Autodesk Inventor part; units mm, degrees
(part 2 of 2)
sketch "Sketch9" plane through (-10, 21.48, -77.0624) normal (0, 0, -1) x (-1, 0, 0)
  line L0 (0.1006, 0.0497) -> (90.0454, 0.0497) construction
  line L1 (90.0454, 0.0497) -> (90.0454, -43.0368) construction
  line L2 (90.0454, -43.0368) -> (0.1006, -43.0368) construction
  line L3 (0.1006, -43.0368) -> (0.1006, 0.0497) construction
  line L4 (5.8424, -17.3579) -> (5.8424, -12.0619)
  line L5 (5.8424, -12.0619) -> (5.6332, -12.0619)
  spline S0 degree 2 poles (5.6332, -12.0619) (5.1253, -12.0619) (4.707, -11.6884) (4.707, -11.3821) knots 0 0 0 1 2 2 2
  spline S1 degree 2 poles (4.707, -11.3821) (4.707, -11.0833) (5.1253, -10.7099) (5.6332, -10.7099) knots 0 0 0 1 2 2 2
  line L6 (5.6332, -10.7099) -> (9.0245, -10.7099)
  spline S2 degree 2 poles (9.0245, -10.7099) (10.2345, -10.7099) (11.7135, -12.0619) (11.7135, -12.9956) knots 0 0 0 1 2 2 2
  spline S3 degree 2 poles (11.7135, -12.9956) (11.7135, -13.4363) (11.3699, -14.2206) (11.0263, -14.5493) knots 0 0 0 1 2 2 2
  spline S4 degree 2 poles (11.0263, -14.5493) (11.6687, -14.9302) (12.3036, -15.9536) (12.3036, -16.596) knots 0 0 0 1 2 2 2
  spline S5 degree 2 poles (12.3036, -16.596) (12.3036, -17.1114) (12.0721, -17.5521) knots 0 0 0 1 1 1
  spline S6 degree 2 poles (12.0721, -17.5521) (11.9003, -17.8882) (11.6538, -18.0824) knots 0 0 0 1 1 1
  spline S7 degree 2 poles (11.6538, -18.0824) (11.3176, -18.3588) (10.3391, -18.7099) (9.6071, -18.7099) knots 0 0 0 1 2 2 2
  line L7 (9.6071, -18.7099) -> (5.6332, -18.7099)
  spline S8 degree 2 poles (5.6332, -18.7099) (5.1253, -18.7099) (4.707, -18.3364) (4.707, -18.0301) knots 0 0 0 1 2 2 2
  spline S9 degree 2 poles (4.707, -18.0301) (4.707, -17.7239) (5.1253, -17.3579) (5.6332, -17.3579) knots 0 0 0 1 2 2 2
  line L8 (5.6332, -17.3579) -> (5.8424, -17.3579)
  line L9 (7.1944, -17.3579) -> (9.5324, -17.3579)
  spline S10 degree 2 poles (9.5324, -17.3579) (10.3541, -17.3579) (10.6977, -17.1114) knots 0 0 0 1 1 1
  spline S11 degree 2 poles (10.6977, -17.1114) (10.9516, -16.9321) (10.9516, -16.5885) knots 0 0 0 1 1 1
  spline S12 degree 2 poles (10.9516, -16.5885) (10.9516, -16.1851) (9.9358, -15.3933) (8.9871, -15.3933) knots 0 0 0 1 2 2 2
  line L10 (8.9871, -15.3933) -> (7.1944, -15.3933)
  line L11 (7.1944, -15.3933) -> (7.1944, -17.3579)
  line L12 (7.1944, -14.0413) -> (8.6809, -14.0413)
  spline S13 degree 2 poles (8.6809, -14.0413) (9.4801, -14.0413) (10.003, -13.638) knots 0 0 0 1 1 1
  spline S14 degree 2 poles (10.003, -13.638) (10.3615, -13.3616) (10.3615, -12.9582) knots 0 0 0 1 1 1
  spline S15 degree 2 poles (10.3615, -12.9582) (10.3615, -12.5997) (9.6893, -12.0619) (8.9572, -12.0619) knots 0 0 0 1 2 2 2
  line L13 (8.9572, -12.0619) -> (7.1944, -12.0619)
  line L14 (7.1944, -12.0619) -> (7.1944, -14.0413)
  line L15 (19.5791, -12.7192) -> (19.5791, -17.3579)
  spline S16 degree 2 poles (19.5791, -17.3579) (20.087, -17.3579) (20.5053, -17.7313) (20.5053, -18.0376) knots 0 0 0 1 2 2 2
  spline S17 degree 2 poles (20.5053, -18.0376) (20.5053, -18.3439) (20.087, -18.7099) (19.5791, -18.7099) knots 0 0 0 1 2 2 2
  line L16 (19.5791, -18.7099) -> (18.2271, -18.7099)
  line L17 (18.2271, -18.7099) -> (18.2271, -18.3961)
  spline S18 degree 2 poles (18.2271, -18.3961) (17.6444, -18.6576) (16.5912, -18.9265) (16.1132, -18.9265) knots 0 0 0 1 2 2 2
  spline S19 degree 2 poles (16.1132, -18.9265) (15.4484, -18.9265) (14.4698, -18.3663) (14.186, -17.8733) knots 0 0 0 1 2 2 2
  spline S20 degree 2 poles (14.186, -17.8733) (13.9843, -17.5147) (13.9843, -16.9769) knots 0 0 0 1 1 1
  line L18 (13.9843, -16.9769) -> (13.9843, -14.0712)
  line L19 (13.9843, -14.0712) -> (13.7528, -14.0712)
  spline S21 degree 2 poles (13.7528, -14.0712) (13.2448, -14.0712) (12.8265, -13.6977) (12.8265, -13.3915) knots 0 0 0 1 2 2 2
  spline S22 degree 2 poles (12.8265, -13.3915) (12.8265, -13.0852) (13.2448, -12.7192) (13.7528, -12.7192) knots 0 0 0 1 2 2 2
  line L20 (13.7528, -12.7192) -> (15.3363, -12.7192)
  line L21 (15.3363, -12.7192) -> (15.3363, -16.7453)
  spline S23 degree 2 poles (15.3363, -16.7453) (15.3363, -17.1711) (15.7546, -17.5745) (16.1804, -17.5745) knots 0 0 0 1 2 2 2
  spline S24 degree 2 poles (16.1804, -17.5745) (16.5912, -17.5745) (17.5324, -17.2533) (18.2271, -16.8275) knots 0 0 0 1 2 2 2
  line L22 (18.2271, -16.8275) -> (18.2271, -14.0712)
  line L23 (18.2271, -14.0712) -> (17.7416, -14.0712)
  spline S25 degree 2 poles (17.7416, -14.0712) (17.2336, -14.0712) (16.8153, -13.6977) (16.8153, -13.3915) knots 0 0 0 1 2 2 2
  spline S26 degree 2 poles (16.8153, -13.3915) (16.8153, -13.0852) (17.2336, -12.7192) (17.7416, -12.7192) knots 0 0 0 1 2 2 2
  line L24 (17.7416, -12.7192) -> (19.5791, -12.7192)
  line L25 (25.4801, -12.7192) -> (25.4801, -17.3579)
  line L26 (25.4801, -17.3579) -> (27.101, -17.3579)
  spline S27 degree 2 poles (27.101, -17.3579) (27.609, -17.3579) (28.0273, -17.7313) (28.0273, -18.0376) knots 0 0 0 1 2 2 2
  spline S28 degree 2 poles (28.0273, -18.0376) (28.0273, -18.3439) (27.609, -18.7099) (27.101, -18.7099) knots 0 0 0 1 2 2 2
  line L27 (27.101, -18.7099) -> (22.5072, -18.7099)
  spline S29 degree 2 poles (22.5072, -18.7099) (21.9993, -18.7099) (21.581, -18.3364) (21.581, -18.0301) knots 0 0 0 1 2 2 2
  spline S30 degree 2 poles (21.581, -18.0301) (21.581, -17.7239) (21.9993, -17.3579) (22.5072, -17.3579) knots 0 0 0 1 2 2 2
  line L28 (22.5072, -17.3579) -> (24.1281, -17.3579)
  line L29 (24.1281, -17.3579) -> (24.1281, -14.0712)
  line L30 (24.1281, -14.0712) -> (23.0375, -14.0712)
  spline S31 degree 2 poles (23.0375, -14.0712) (22.5296, -14.0712) (22.1113, -13.6977) (22.1113, -13.3915) knots 0 0 0 1 2 2 2
  spline S32 degree 2 poles (22.1113, -13.3915) (22.1113, -13.0852) (22.5296, -12.7192) (23.0375, -12.7192) knots 0 0 0 1 2 2 2
  line L31 (23.0375, -12.7192) -> (25.4801, -12.7192)
  line L32 (25.2934, -10.1571) -> (25.2934, -11.5913)
  line L33 (25.2934, -11.5913) -> (23.6874, -11.5913)
  line L34 (23.6874, -11.5913) -> (23.6874, -10.1571)
  line L35 (23.6874, -10.1571) -> (25.2934, -10.1571)
  line L36 (33.5847, -10.1571) -> (33.5847, -17.3579)
  line L37 (33.5847, -17.3579) -> (35.2056, -17.3579)
  spline S33 degree 2 poles (35.2056, -17.3579) (35.7135, -17.3579) (36.1318, -17.7313) (36.1318, -18.0376) knots 0 0 0 1 2 2 2
  spline S34 degree 2 poles (36.1318, -18.0376) (36.1318, -18.3439) (35.7135, -18.7099) (35.2056, -18.7099) knots 0 0 0 1 2 2 2
  line L38 (35.2056, -18.7099) -> (30.6118, -18.7099)
  spline S35 degree 2 poles (30.6118, -18.7099) (30.1038, -18.7099) (29.6855, -18.3364) (29.6855, -18.0301) knots 0 0 0 1 2 2 2
  spline S36 degree 2 poles (29.6855, -18.0301) (29.6855, -17.7239) (30.1038, -17.3579) (30.6118, -17.3579) knots 0 0 0 1 2 2 2
  line L39 (30.6118, -17.3579) -> (32.2327, -17.3579)
  line L40 (32.2327, -17.3579) -> (32.2327, -11.5091)
  line L41 (32.2327, -11.5091) -> (31.1421, -11.5091)
  spline S37 degree 2 poles (31.1421, -11.5091) (30.6342, -11.5091) (30.2159, -11.1356) (30.2159, -10.8294) knots 0 0 0 1 2 2 2
  spline S38 degree 2 poles (30.2159, -10.8294) (30.2159, -10.5231) (30.6342, -10.1571) (31.1421, -10.1571) knots 0 0 0 1 2 2 2
  line L42 (31.1421, -10.1571) -> (33.5847, -10.1571)
  line L43 (44.1169, -10.1571) -> (44.1169, -17.3579)
  line L44 (44.1169, -17.3579) -> (44.3485, -17.3579)
  spline S39 degree 2 poles (44.3485, -17.3579) (44.8564, -17.3579) (45.2747, -17.7313) (45.2747, -18.0376) knots 0 0 0 1 2 2 2
  spline S40 degree 2 poles (45.2747, -18.0376) (45.2747, -18.3439) (44.8564, -18.7099) (44.3485, -18.7099) knots 0 0 0 1 2 2 2
  line L45 (44.3485, -18.7099) -> (42.7649, -18.7099)
  line L46 (42.7649, -18.7099) -> (42.7649, -18.3812)
  spline S41 degree 2 poles (42.7649, -18.3812) (42.3018, -18.6501) (41.2934, -18.9265) (40.7556, -18.9265) knots 0 0 0 1 2 2 2
  spline S42 degree 2 poles (40.7556, -18.9265) (39.2392, -18.9265) (37.3793, -17.1636) (37.3793, -15.8565) knots 0 0 0 1 2 2 2
  spline S43 degree 2 poles (37.3793, -15.8565) (37.3793, -14.482) (39.3289, -12.5474) (40.7331, -12.5474) knots 0 0 0 1 2 2 2
  spline S44 degree 2 poles (40.7331, -12.5474) (41.256, -12.5474) (42.2719, -12.8686) (42.7649, -13.1973) knots 0 0 0 1 2 2 2
  line L47 (42.7649, -13.1973) -> (42.7649, -11.5091)
  line L48 (42.7649, -11.5091) -> (42.5333, -11.5091)
  spline S45 degree 2 poles (42.5333, -11.5091) (42.0254, -11.5091) (41.6071, -11.1431) (41.6071, -10.8368) knots 0 0 0 1 2 2 2
  spline S46 degree 2 poles (41.6071, -10.8368) (41.6071, -10.5306) (42.0254, -10.1571) (42.5333, -10.1571) knots 0 0 0 1 2 2 2
  line L49 (42.5333, -10.1571) -> (44.1169, -10.1571)
  spline S47 degree 2 poles (42.7649, -15.8938) (42.7649, -15.0572) (41.5922, -13.8994) (40.7481, -13.8994) knots 0 0 0 1 2 2 2
  spline S48 degree 2 poles (40.7481, -13.8994) (39.904, -13.8994) (38.7313, -15.0572) (38.7313, -15.8789) knots 0 0 0 1 2 2 2
  spline S49 degree 2 poles (38.7313, -15.8789) (38.7313, -16.6184) (39.7845, -17.5745) (40.7481, -17.5745) knots 0 0 0 1 2 2 2
  spline S50 degree 2 poles (40.7481, -17.5745) (41.6967, -17.5745) (42.7649, -16.6184) (42.7649, -15.8938) knots 0 0 0 1 2 2 2
  line L50 (50.3391, -18.7099) -> (50.3391, -18.3961)
  spline S51 degree 2 poles (50.3391, -18.3961) (49.8312, -18.6576) (48.6062, -18.9265) (48.1057, -18.9265) knots 0 0 0 1 2 2 2
  spline S52 degree 2 poles (48.1057, -18.9265) (47.0226, -18.9265) (45.6631, -17.7762) (45.6631, -17.0815) knots 0 0 0 1 2 2 2
  spline S53 degree 2 poles (45.6631, -17.0815) (45.6631, -16.2299) (47.3961, -14.7808) (48.9199, -14.7808) knots 0 0 0 1 2 2 2
  spline S54 degree 2 poles (48.9199, -14.7808) (49.5324, -14.7808) (50.3391, -14.9153) knots 0 0 0 1 1 1
  line L51 (50.3391, -14.9153) -> (50.3391, -14.5866)
  spline S55 degree 2 poles (50.3391, -14.5866) (50.3391, -14.2804) (49.8162, -13.8994) (49.0917, -13.8994) knots 0 0 0 1 2 2 2
  spline S56 degree 2 poles (49.0917, -13.8994) (48.4866, -13.8994) (47.5305, -14.1384) knots 0 0 0 1 1 1
  spline S57 degree 2 poles (47.5305, -14.1384) (47.1795, -14.2206) (46.9778, -14.2206) knots 0 0 0 1 1 1
  spline S58 degree 2 poles (46.9778, -14.2206) (46.7089, -14.2206) (46.3354, -13.8322) (46.3354, -13.5259) knots 0 0 0 1 2 2 2
  spline S59 degree 2 poles (46.3354, -13.5259) (46.3354, -13.3541) (46.4698, -13.1076) (46.7014, -12.9582) (47.0824, -12.8537) knots 0 0 0 1 2 3 3 3
  spline S60 degree 2 poles (47.0824, -12.8537) (47.5828, -12.7117) (48.6211, -12.5474) (49.0394, -12.5474) knots 0 0 0 1 2 2 2
  spline S61 degree 2 poles (49.0394, -12.5474) (50.3018, -12.5474) (51.6911, -13.638) (51.6911, -14.5791) knots 0 0 0 1 2 2 2
  line L52 (51.6911, -14.5791) -> (51.6911, -17.3579)
  line L53 (51.6911, -17.3579) -> (51.9227, -17.3579)
  spline S62 degree 2 poles (51.9227, -17.3579) (52.4306, -17.3579) (52.8489, -17.7313) (52.8489, -18.0376) knots 0 0 0 1 2 2 2
  spline S63 degree 2 poles (52.8489, -18.0376) (52.8489, -18.3439) (52.4306, -18.7099) (51.9227, -18.7099) knots 0 0 0 1 2 2 2
  line L54 (51.9227, -18.7099) -> (50.3391, -18.7099)
  spline S64 degree 2 poles (50.3391, -16.2897) (49.5324, -16.1328) (48.8452, -16.1328) knots 0 0 0 1 1 1
  spline S65 degree 2 poles (48.8452, -16.1328) (48.0235, -16.1328) (47.426, -16.5362) knots 0 0 0 1 1 1
  spline S66 degree 2 poles (47.426, -16.5362) (47.0599, -16.7902) (47.0599, -17.0516) knots 0 0 0 1 1 1
  spline S67 degree 2 poles (47.0599, -17.0516) (47.0599, -17.2383) (47.2392, -17.3579) knots 0 0 0 1 1 1
  spline S68 degree 2 poles (47.2392, -17.3579) (47.5679, -17.5745) (48.143, -17.5745) knots 0 0 0 1 1 1
  spline S69 degree 2 poles (48.143, -17.5745) (48.6286, -17.5745) (49.8611, -17.1935) (50.3391, -16.8649) knots 0 0 0 1 2 2 2
  line L55 (50.3391, -16.8649) -> (50.3391, -16.2897)
  line L56 (55.5231, -10.1571) -> (55.5231, -13.1973)
  spline S70 degree 2 poles (55.5231, -13.1973) (56.0161, -12.8686) (57.0394, -12.5474) (57.5623, -12.5474) knots 0 0 0 1 2 2 2
  spline S71 degree 2 poles (57.5623, -12.5474) (58.9666, -12.5474) (60.9162, -14.482) (60.9162, -15.8565) knots 0 0 0 1 2 2 2
  spline S72 degree 2 poles (60.9162, -15.8565) (60.9162, -17.1636) (59.0562, -18.9265) (57.5324, -18.9265) knots 0 0 0 1 2 2 2
  spline S73 degree 2 poles (57.5324, -18.9265) (56.9946, -18.9265) (55.9937, -18.6501) (55.5231, -18.3737) knots 0 0 0 1 2 2 2
  line L57 (55.5231, -18.3737) -> (55.5231, -18.7099)
  line L58 (55.5231, -18.7099) -> (53.9395, -18.7099)
  spline S74 degree 2 poles (53.9395, -18.7099) (53.4316, -18.7099) (53.0133, -18.3364) (53.0133, -18.0301) knots 0 0 0 1 2 2 2
  spline S75 degree 2 poles (53.0133, -18.0301) (53.0133, -17.7239) (53.4316, -17.3579) (53.9395, -17.3579) knots 0 0 0 1 2 2 2
  line L59 (53.9395, -17.3579) -> (54.1711, -17.3579)
  line L60 (54.1711, -17.3579) -> (54.1711, -11.5091)
  line L61 (54.1711, -11.5091) -> (53.9395, -11.5091)
  spline S76 degree 2 poles (53.9395, -11.5091) (53.4316, -11.5091) (53.0133, -11.1356) (53.0133, -10.8294) knots 0 0 0 1 2 2 2
  spline S77 degree 2 poles (53.0133, -10.8294) (53.0133, -10.5231) (53.4316, -10.1571) (53.9395, -10.1571) knots 0 0 0 1 2 2 2
  line L62 (53.9395, -10.1571) -> (55.5231, -10.1571)
  spline S78 degree 2 poles (59.5641, -15.8938) (59.5641, -15.0572) (58.3914, -13.8994) (57.5399, -13.8994) knots 0 0 0 1 2 2 2
  spline S79 degree 2 poles (57.5399, -13.8994) (56.6958, -13.8994) (55.5231, -15.0572) (55.5231, -15.8789) knots 0 0 0 1 2 2 2
  spline S80 degree 2 poles (55.5231, -15.8789) (55.5231, -16.6184) (56.5763, -17.5745) (57.5399, -17.5745) knots 0 0 0 1 2 2 2
  spline S81 degree 2 poles (57.5399, -17.5745) (58.5035, -17.5745) (59.5641, -16.6184) (59.5641, -15.8938) knots 0 0 0 1 2 2 2
  line L63 (66.003, -10.1571) -> (66.003, -17.3579)
  line L64 (66.003, -17.3579) -> (67.6239, -17.3579)
  spline S82 degree 2 poles (67.6239, -17.3579) (68.1318, -17.3579) (68.5501, -17.7313) (68.5501, -18.0376) knots 0 0 0 1 2 2 2
  spline S83 degree 2 poles (68.5501, -18.0376) (68.5501, -18.3439) (68.1318, -18.7099) (67.6239, -18.7099) knots 0 0 0 1 2 2 2
  line L65 (67.6239, -18.7099) -> (63.0301, -18.7099)
  spline S84 degree 2 poles (63.0301, -18.7099) (62.5221, -18.7099) (62.1038, -18.3364) (62.1038, -18.0301) knots 0 0 0 1 2 2 2
  spline S85 degree 2 poles (62.1038, -18.0301) (62.1038, -17.7239) (62.5221, -17.3579) (63.0301, -17.3579) knots 0 0 0 1 2 2 2
  line L66 (63.0301, -17.3579) -> (64.651, -17.3579)
  line L67 (64.651, -17.3579) -> (64.651, -11.5091)
  line L68 (64.651, -11.5091) -> (63.5604, -11.5091)
  spline S86 degree 2 poles (63.5604, -11.5091) (63.0525, -11.5091) (62.6342, -11.1356) (62.6342, -10.8294) knots 0 0 0 1 2 2 2
  spline S87 degree 2 poles (62.6342, -10.8294) (62.6342, -10.5231) (63.0525, -10.1571) (63.5604, -10.1571) knots 0 0 0 1 2 2 2
  line L69 (63.5604, -10.1571) -> (66.003, -10.1571)
  line L70 (76.834, -16.4017) -> (71.284, -16.4017)
  spline S88 degree 2 poles (71.284, -16.4017) (71.4932, -16.9321) (72.5688, -17.5745) (73.4876, -17.5745) knots 0 0 0 1 2 2 2
  spline S89 degree 2 poles (73.4876, -17.5745) (74.242, -17.5745) (75.4895, -17.2533) knots 0 0 0 1 1 1
  spline S90 degree 2 poles (75.4895, -17.2533) (76.0049, -17.1188) (76.1991, -17.1188) knots 0 0 0 1 1 1
  spline S91 degree 2 poles (76.1991, -17.1188) (76.4754, -17.1188) (76.8415, -17.4998) (76.8415, -17.7911) knots 0 0 0 1 2 2 2
  spline S92 degree 2 poles (76.8415, -17.7911) (76.8415, -18.0525) (76.6472, -18.2393) knots 0 0 0 1 1 1
  spline S93 degree 2 poles (76.6472, -18.2393) (76.3783, -18.4858) (74.3317, -18.9265) (73.3905, -18.9265) knots 0 0 0 1 2 2 2
  spline S94 degree 2 poles (73.3905, -18.9265) (71.7696, -18.9265) (69.82, -17.0964) (69.82, -15.7594) knots 0 0 0 1 2 2 2
  spline S95 degree 2 poles (69.82, -15.7594) (69.82, -14.3326) (71.9264, -12.5474) (73.3008, -12.5474) knots 0 0 0 1 2 2 2
  spline S96 degree 2 poles (73.3008, -12.5474) (74.1225, -12.5474) (75.5044, -13.13) (75.8405, -13.4662) knots 0 0 0 1 2 2 2
  spline S97 degree 2 poles (75.8405, -13.4662) (76.3111, -13.9517) (76.6248, -14.6688) knots 0 0 0 1 1 1
  spline S98 degree 2 poles (76.6248, -14.6688) (76.834, -15.1692) (76.834, -15.8266) knots 0 0 0 1 1 1
  line L71 (76.834, -15.8266) -> (76.834, -16.4017)
  spline S99 degree 2 poles (75.3401, -15.0497) (75.0263, -14.4746) (74.0254, -13.8994) (73.3307, -13.8994) knots 0 0 0 1 2 2 2
  spline S100 degree 2 poles (73.3307, -13.8994) (72.6435, -13.8994) (71.6351, -14.4746) (71.3214, -15.0497) knots 0 0 0 1 2 2 2
  line L72 (71.3214, -15.0497) -> (75.3401, -15.0497)
  line L73 (13.947, -31.2614) -> (13.947, -25.9654)
  line L74 (13.947, -25.9654) -> (13.7378, -25.9654)
  spline S101 degree 2 poles (13.7378, -25.9654) (13.2299, -25.9654) (12.8116, -25.5919) (12.8116, -25.2857) knots 0 0 0 1 2 2 2
  spline S102 degree 2 poles (12.8116, -25.2857) (12.8116, -24.9869) (13.2299, -24.6134) (13.7378, -24.6134) knots 0 0 0 1 2 2 2
  line L75 (13.7378, -24.6134) -> (17.129, -24.6134)
  spline S103 degree 2 poles (17.129, -24.6134) (18.3391, -24.6134) (19.8181, -25.9654) (19.8181, -26.8991) knots 0 0 0 1 2 2 2
  spline S104 degree 2 poles (19.8181, -26.8991) (19.8181, -27.3398) (19.4745, -28.1242) (19.1309, -28.4528) knots 0 0 0 1 2 2 2
  spline S105 degree 2 poles (19.1309, -28.4528) (19.7733, -28.8338) (20.4082, -29.8571) (20.4082, -30.4995) knots 0 0 0 1 2 2 2
  spline S106 degree 2 poles (20.4082, -30.4995) (20.4082, -31.0149) (20.1767, -31.4556) knots 0 0 0 1 1 1
  spline S107 degree 2 poles (20.1767, -31.4556) (20.0049, -31.7918) (19.7584, -31.986) knots 0 0 0 1 1 1
  spline S108 degree 2 poles (19.7584, -31.986) (19.4222, -32.2624) (18.4437, -32.6134) (17.7117, -32.6134) knots 0 0 0 1 2 2 2
  line L76 (17.7117, -32.6134) -> (13.7378, -32.6134)
  spline S109 degree 2 poles (13.7378, -32.6134) (13.2299, -32.6134) (12.8116, -32.2399) (12.8116, -31.9337) knots 0 0 0 1 2 2 2
  spline S110 degree 2 poles (12.8116, -31.9337) (12.8116, -31.6274) (13.2299, -31.2614) (13.7378, -31.2614) knots 0 0 0 1 2 2 2
  line L77 (13.7378, -31.2614) -> (13.947, -31.2614)
  line L78 (15.299, -31.2614) -> (17.637, -31.2614)
  spline S111 degree 2 poles (17.637, -31.2614) (18.4586, -31.2614) (18.8022, -31.0149) knots 0 0 0 1 1 1
  spline S112 degree 2 poles (18.8022, -31.0149) (19.0562, -30.8356) (19.0562, -30.492) knots 0 0 0 1 1 1
  spline S113 degree 2 poles (19.0562, -30.492) (19.0562, -30.0887) (18.0403, -29.2969) (17.0917, -29.2969) knots 0 0 0 1 2 2 2
  line L79 (17.0917, -29.2969) -> (15.299, -29.2969)
  line L80 (15.299, -29.2969) -> (15.299, -31.2614)
  line L81 (15.299, -27.9449) -> (16.7854, -27.9449)
  spline S114 degree 2 poles (16.7854, -27.9449) (17.5847, -27.9449) (18.1076, -27.5415) knots 0 0 0 1 1 1
  spline S115 degree 2 poles (18.1076, -27.5415) (18.4661, -27.2652) (18.4661, -26.8618) knots 0 0 0 1 1 1
  spline S116 degree 2 poles (18.4661, -26.8618) (18.4661, -26.5032) (17.7938, -25.9654) (17.0618, -25.9654) knots 0 0 0 1 2 2 2
  line L82 (17.0618, -25.9654) -> (15.299, -25.9654)
  line L83 (15.299, -25.9654) -> (15.299, -27.9449)
  line L84 (26.0254, -32.6134) -> (26.0254, -32.2997)
  spline S117 degree 2 poles (26.0254, -32.2997) (25.5175, -32.5611) (24.2924, -32.83) (23.792, -32.83) knots 0 0 0 1 2 2 2
  spline S118 degree 2 poles (23.792, -32.83) (22.7089, -32.83) (21.3494, -31.6797) (21.3494, -30.985) knots 0 0 0 1 2 2 2
  spline S119 degree 2 poles (21.3494, -30.985) (21.3494, -30.1335) (23.0824, -28.6844) (24.6062, -28.6844) knots 0 0 0 1 2 2 2
  spline S120 degree 2 poles (24.6062, -28.6844) (25.2187, -28.6844) (26.0254, -28.8188) knots 0 0 0 1 1 1
  line L85 (26.0254, -28.8188) -> (26.0254, -28.4902)
  spline S121 degree 2 poles (26.0254, -28.4902) (26.0254, -28.1839) (25.5025, -27.803) (24.778, -27.803) knots 0 0 0 1 2 2 2
  spline S122 degree 2 poles (24.778, -27.803) (24.1729, -27.803) (23.2168, -28.042) knots 0 0 0 1 1 1
  spline S123 degree 2 poles (23.2168, -28.042) (22.8657, -28.1242) (22.6641, -28.1242) knots 0 0 0 1 1 1
  spline S124 degree 2 poles (22.6641, -28.1242) (22.3951, -28.1242) (22.0217, -27.7357) (22.0217, -27.4295) knots 0 0 0 1 2 2 2
  spline S125 degree 2 poles (22.0217, -27.4295) (22.0217, -27.2577) (22.1561, -27.0112) (22.3877, -26.8618) (22.7686, -26.7572) knots 0 0 0 1 2 3 3 3
  spline S126 degree 2 poles (22.7686, -26.7572) (23.2691, -26.6153) (24.3074, -26.451) (24.7257, -26.451) knots 0 0 0 1 2 2 2
  spline S127 degree 2 poles (24.7257, -26.451) (25.988, -26.451) (27.3774, -27.5415) (27.3774, -28.4827) knots 0 0 0 1 2 2 2
  line L86 (27.3774, -28.4827) -> (27.3774, -31.2614)
  line L87 (27.3774, -31.2614) -> (27.609, -31.2614)
  spline S128 degree 2 poles (27.609, -31.2614) (28.1169, -31.2614) (28.5352, -31.6349) (28.5352, -31.9412) knots 0 0 0 1 2 2 2
  spline S129 degree 2 poles (28.5352, -31.9412) (28.5352, -32.2474) (28.1169, -32.6134) (27.609, -32.6134) knots 0 0 0 1 2 2 2
  line L88 (27.609, -32.6134) -> (26.0254, -32.6134)
  spline S130 degree 2 poles (26.0254, -30.1933) (25.2187, -30.0364) (24.5315, -30.0364) knots 0 0 0 1 1 1
  spline S131 degree 2 poles (24.5315, -30.0364) (23.7098, -30.0364) (23.1122, -30.4398) knots 0 0 0 1 1 1
  spline S132 degree 2 poles (23.1122, -30.4398) (22.7462, -30.6937) (22.7462, -30.9552) knots 0 0 0 1 1 1
  spline S133 degree 2 poles (22.7462, -30.9552) (22.7462, -31.1419) (22.9255, -31.2614) knots 0 0 0 1 1 1
  spline S134 degree 2 poles (22.9255, -31.2614) (23.2542, -31.478) (23.8293, -31.478) knots 0 0 0 1 1 1
  spline S135 degree 2 poles (23.8293, -31.478) (24.3148, -31.478) (25.5473, -31.0971) (26.0254, -30.7684) knots 0 0 0 1 2 2 2
  line L89 (26.0254, -30.7684) -> (26.0254, -30.1933)
  spline S136 degree 2 poles (35.0263, -26.8767) (35.2654, -26.6377) (35.5268, -26.6377) knots 0 0 0 1 1 1
  spline S137 degree 2 poles (35.5268, -26.6377) (35.8181, -26.6377) (36.1916, -27.056) (36.1916, -27.5341) knots 0 0 0 1 2 2 2
  line L90 (36.1916, -27.5341) -> (36.1916, -28.408)
  spline S138 degree 2 poles (36.1916, -28.408) (36.1916, -28.8935) (35.8181, -29.3044) (35.5119, -29.3044) knots 0 0 0 1 2 2 2
  spline S139 degree 2 poles (35.5119, -29.3044) (35.2355, -29.3044) (35.0413, -29.1475) knots 0 0 0 1 1 1
  spline S140 degree 2 poles (35.0413, -29.1475) (34.9068, -29.028) (34.75, -28.296) (34.4437, -28.1167) knots 0 0 0 1 2 2 2
  spline S141 degree 2 poles (34.4437, -28.1167) (33.9134, -27.803) (33.0768, -27.803) knots 0 0 0 1 1 1
  spline S142 degree 2 poles (33.0768, -27.803) (32.1206, -27.803) (30.9703, -28.9234) (30.9703, -29.775) knots 0 0 0 1 2 2 2
  spline S143 degree 2 poles (30.9703, -29.775) (30.9703, -30.5667) (32.0758, -31.478) (33.3606, -31.478) knots 0 0 0 1 2 2 2
  spline S144 degree 2 poles (33.3606, -31.478) (34.2047, -31.478) (34.7425, -31.3062) knots 0 0 0 1 1 1
  spline S145 degree 2 poles (34.7425, -31.3062) (35.0562, -31.2017) (35.6239, -30.6937) (35.8555, -30.6937) knots 0 0 0 1 2 2 2
  spline S146 degree 2 poles (35.8555, -30.6937) (36.1318, -30.6937) (36.5352, -31.1046) (36.5352, -31.3809) knots 0 0 0 1 2 2 2
  spline S147 degree 2 poles (36.5352, -31.3809) (36.5352, -31.8291) (35.9227, -32.2325) knots 0 0 0 1 1 1
  spline S148 degree 2 poles (35.9227, -32.2325) (35.0114, -32.83) (33.256, -32.83) knots 0 0 0 1 1 1
  spline S149 degree 2 poles (33.256, -32.83) (31.6799, -32.83) (30.806, -32.1802) knots 0 0 0 1 1 1
  spline S150 degree 2 poles (30.806, -32.1802) (29.6183, -31.3062) (29.6183, -29.7824) knots 0 0 0 1 1 1
  spline S151 degree 2 poles (29.6183, -29.7824) (29.6183, -28.3408) (31.5455, -26.451) (33.0917, -26.451) knots 0 0 0 1 2 2 2
  spline S152 degree 2 poles (33.0917, -26.451) (33.6519, -26.451) (34.6155, -26.6601) (35.0263, -26.8767) knots 0 0 0 1 2 2 2
  line L91 (40.6883, -27.9748) -> (40.6883, -30.6863)
  spline S153 degree 2 poles (40.6883, -30.6863) (40.6883, -31.1195) (40.8676, -31.2614) knots 0 0 0 1 1 1
  spline S154 degree 2 poles (40.8676, -31.2614) (41.144, -31.478) (41.8536, -31.478) knots 0 0 0 1 1 1
  spline S155 degree 2 poles (41.8536, -31.478) (42.8919, -31.478) (43.7658, -31.0373) knots 0 0 0 1 1 1
  spline S156 degree 2 poles (43.7658, -31.0373) (44.102, -30.8655) (44.2962, -30.8655) knots 0 0 0 1 1 1
  spline S157 degree 2 poles (44.2962, -30.8655) (44.5576, -30.8655) (44.946, -31.2614) (44.946, -31.5453) knots 0 0 0 1 2 2 2
  spline S158 degree 2 poles (44.946, -31.5453) (44.946, -31.8067) (44.7369, -32.0009) knots 0 0 0 1 1 1
  spline S159 degree 2 poles (44.7369, -32.0009) (44.4157, -32.3072) (42.5035, -32.83) (41.8536, -32.83) knots 0 0 0 1 2 2 2
  spline S160 degree 2 poles (41.8536, -32.83) (40.5987, -32.83) (39.3363, -31.7395) (39.3363, -30.9477) knots 0 0 0 1 2 2 2
  line L92 (39.3363, -30.9477) -> (39.3363, -27.9748)
  line L93 (39.3363, -27.9748) -> (38.8508, -27.9748)
  spline S161 degree 2 poles (38.8508, -27.9748) (38.3653, -27.9748) (37.947, -27.6013) (37.947, -27.295) knots 0 0 0 1 2 2 2
  spline S162 degree 2 poles (37.947, -27.295) (37.947, -26.9962) (38.3653, -26.6228) (38.8508, -26.6228) knots 0 0 0 1 2 2 2
  line L94 (38.8508, -26.6228) -> (39.3363, -26.6228)
  line L95 (39.3363, -26.6228) -> (39.3363, -25.4052)
  spline S163 degree 2 poles (39.3363, -25.4052) (39.3363, -24.9197) (39.7098, -24.5014) (40.0161, -24.5014) knots 0 0 0 1 2 2 2
  spline S164 degree 2 poles (40.0161, -24.5014) (40.3148, -24.5014) (40.6883, -24.9197) (40.6883, -25.4052) knots 0 0 0 1 2 2 2
  line L96 (40.6883, -25.4052) -> (40.6883, -26.6228)
  line L97 (40.6883, -26.6228) -> (43.1832, -26.6228)
  spline S165 degree 2 poles (43.1832, -26.6228) (43.6687, -26.6228) (44.087, -26.9962) (44.087, -27.3025) knots 0 0 0 1 2 2 2
  spline S166 degree 2 poles (44.087, -27.3025) (44.087, -27.6013) (43.6687, -27.9748) (43.1832, -27.9748) knots 0 0 0 1 2 2 2
  line L98 (43.1832, -27.9748) -> (40.6883, -27.9748)
  line L99 (52.5203, -30.3053) -> (46.9703, -30.3053)
  spline S167 degree 2 poles (46.9703, -30.3053) (47.1795, -30.8356) (48.2551, -31.478) (49.1739, -31.478) knots 0 0 0 1 2 2 2
  spline S168 degree 2 poles (49.1739, -31.478) (49.9283, -31.478) (51.1757, -31.1568) knots 0 0 0 1 1 1
  spline S169 degree 2 poles (51.1757, -31.1568) (51.6911, -31.0224) (51.8853, -31.0224) knots 0 0 0 1 1 1
  spline S170 degree 2 poles (51.8853, -31.0224) (52.1617, -31.0224) (52.5277, -31.4033) (52.5277, -31.6947) knots 0 0 0 1 2 2 2
  spline S171 degree 2 poles (52.5277, -31.6947) (52.5277, -31.9561) (52.3335, -32.1428) knots 0 0 0 1 1 1
  spline S172 degree 2 poles (52.3335, -32.1428) (52.0646, -32.3893) (50.0179, -32.83) (49.0768, -32.83) knots 0 0 0 1 2 2 2
  spline S173 degree 2 poles (49.0768, -32.83) (47.4558, -32.83) (45.5063, -31) (45.5063, -29.6629) knots 0 0 0 1 2 2 2
  spline S174 degree 2 poles (45.5063, -29.6629) (45.5063, -28.2362) (47.6127, -26.451) (48.9871, -26.451) knots 0 0 0 1 2 2 2
  spline S175 degree 2 poles (48.9871, -26.451) (49.8088, -26.451) (51.1907, -27.0336) (51.5268, -27.3697) knots 0 0 0 1 2 2 2
  spline S176 degree 2 poles (51.5268, -27.3697) (51.9974, -27.8553) (52.3111, -28.5723) knots 0 0 0 1 1 1
  spline S177 degree 2 poles (52.3111, -28.5723) (52.5203, -29.0728) (52.5203, -29.7301) knots 0 0 0 1 1 1
  line L100 (52.5203, -29.7301) -> (52.5203, -30.3053)
  spline S178 degree 2 poles (51.0263, -28.9533) (50.7126, -28.3781) (49.7117, -27.803) (49.017, -27.803) knots 0 0 0 1 2 2 2
  spline S179 degree 2 poles (49.017, -27.803) (48.3298, -27.803) (47.3214, -28.3781) (47.0077, -28.9533) knots 0 0 0 1 2 2 2
  line L101 (47.0077, -28.9533) -> (51.0263, -28.9533)
  line L102 (56.9498, -26.6228) -> (56.9498, -27.4743)
  spline S180 degree 2 poles (56.9498, -27.4743) (57.8013, -26.8618) (58.7873, -26.451) (59.2131, -26.451) knots 0 0 0 1 2 2 2
  spline S181 degree 2 poles (59.2131, -26.451) (59.8704, -26.451) (60.4904, -26.9365) knots 0 0 0 1 1 1
  spline S182 degree 2 poles (60.4904, -26.9365) (60.9162, -27.2652) (60.9162, -27.6088) knots 0 0 0 1 1 1
  spline S183 degree 2 poles (60.9162, -27.6088) (60.9162, -27.9001) (60.5128, -28.3034) (60.2289, -28.3034) knots 0 0 0 1 2 2 2
  spline S184 degree 2 poles (60.2289, -28.3034) (59.9824, -28.3034) (59.4222, -27.803) (59.2056, -27.803) knots 0 0 0 1 2 2 2
  spline S185 degree 2 poles (59.2056, -27.803) (58.9218, -27.803) (57.7938, -28.5126) (56.9498, -29.2297) knots 0 0 0 1 2 2 2
  line L103 (56.9498, -29.2297) -> (56.9498, -31.2614)
  line L104 (56.9498, -31.2614) -> (58.8769, -31.2614)
  spline S186 degree 2 poles (58.8769, -31.2614) (59.3849, -31.2614) (59.8032, -31.6349) (59.8032, -31.9412) knots 0 0 0 1 2 2 2
  spline S187 degree 2 poles (59.8032, -31.9412) (59.8032, -32.2474) (59.3849, -32.6134) (58.8769, -32.6134) knots 0 0 0 1 2 2 2
  line L105 (58.8769, -32.6134) -> (54.791, -32.6134)
  spline S188 degree 2 poles (54.791, -32.6134) (54.2831, -32.6134) (53.8648, -32.2399) (53.8648, -31.9337) knots 0 0 0 1 2 2 2
  spline S189 degree 2 poles (53.8648, -31.9337) (53.8648, -31.6274) (54.2831, -31.2614) (54.791, -31.2614) knots 0 0 0 1 2 2 2
  line L106 (54.791, -31.2614) -> (55.5978, -31.2614)
  line L107 (55.5978, -31.2614) -> (55.5978, -27.9748)
  line L108 (55.5978, -27.9748) -> (55.1122, -27.9748)
  spline S190 degree 2 poles (55.1122, -27.9748) (54.6043, -27.9748) (54.186, -27.6013) (54.186, -27.295) knots 0 0 0 1 2 2 2
  spline S191 degree 2 poles (54.186, -27.295) (54.186, -26.9888) (54.6043, -26.6228) (55.1122, -26.6228) knots 0 0 0 1 2 2 2
  line L109 (55.1122, -26.6228) -> (56.9498, -26.6228)
  line L110 (66.003, -26.6228) -> (66.003, -31.2614)
  line L111 (66.003, -31.2614) -> (67.6239, -31.2614)
  spline S192 degree 2 poles (67.6239, -31.2614) (68.1318, -31.2614) (68.5501, -31.6349) (68.5501, -31.9412) knots 0 0 0 1 2 2 2
  spline S193 degree 2 poles (68.5501, -31.9412) (68.5501, -32.2474) (68.1318, -32.6134) (67.6239, -32.6134) knots 0 0 0 1 2 2 2
  line L112 (67.6239, -32.6134) -> (63.0301, -32.6134)
  spline S194 degree 2 poles (63.0301, -32.6134) (62.5221, -32.6134) (62.1038, -32.2399) (62.1038, -31.9337) knots 0 0 0 1 2 2 2
  spline S195 degree 2 poles (62.1038, -31.9337) (62.1038, -31.6274) (62.5221, -31.2614) (63.0301, -31.2614) knots 0 0 0 1 2 2 2
  line L113 (63.0301, -31.2614) -> (64.651, -31.2614)
  line L114 (64.651, -31.2614) -> (64.651, -27.9748)
  line L115 (64.651, -27.9748) -> (63.5604, -27.9748)
  spline S196 degree 2 poles (63.5604, -27.9748) (63.0525, -27.9748) (62.6342, -27.6013) (62.6342, -27.295) knots 0 0 0 1 2 2 2
  spline S197 degree 2 poles (62.6342, -27.295) (62.6342, -26.9888) (63.0525, -26.6228) (63.5604, -26.6228) knots 0 0 0 1 2 2 2
  line L116 (63.5604, -26.6228) -> (66.003, -26.6228)
  line L117 (65.8162, -24.0607) -> (65.8162, -25.4948)
  line L118 (65.8162, -25.4948) -> (64.2103, -25.4948)
  line L119 (64.2103, -25.4948) -> (64.2103, -24.0607)
  line L120 (64.2103, -24.0607) -> (65.8162, -24.0607)
  line L121 (74.6528, -32.6134) -> (74.6528, -32.2997)
  spline S198 degree 2 poles (74.6528, -32.2997) (74.1449, -32.5611) (72.9199, -32.83) (72.4194, -32.83) knots 0 0 0 1 2 2 2
  spline S199 degree 2 poles (72.4194, -32.83) (71.3363, -32.83) (69.9768, -31.6797) (69.9768, -30.985) knots 0 0 0 1 2 2 2
  spline S200 degree 2 poles (69.9768, -30.985) (69.9768, -30.1335) (71.7098, -28.6844) (73.2336, -28.6844) knots 0 0 0 1 2 2 2
  spline S201 degree 2 poles (73.2336, -28.6844) (73.8461, -28.6844) (74.6528, -28.8188) knots 0 0 0 1 1 1
  line L122 (74.6528, -28.8188) -> (74.6528, -28.4902)
  spline S202 degree 2 poles (74.6528, -28.4902) (74.6528, -28.1839) (74.13, -27.803) (73.4054, -27.803) knots 0 0 0 1 2 2 2
  spline S203 degree 2 poles (73.4054, -27.803) (72.8004, -27.803) (71.8443, -28.042) knots 0 0 0 1 1 1
  spline S204 degree 2 poles (71.8443, -28.042) (71.4932, -28.1242) (71.2915, -28.1242) knots 0 0 0 1 1 1
  spline S205 degree 2 poles (71.2915, -28.1242) (71.0226, -28.1242) (70.6491, -27.7357) (70.6491, -27.4295) knots 0 0 0 1 2 2 2
  spline S206 degree 2 poles (70.6491, -27.4295) (70.6491, -27.2577) (70.7836, -27.0112) (71.0151, -26.8618) (71.3961, -26.7572) knots 0 0 0 1 2 3 3 3
  spline S207 degree 2 poles (71.3961, -26.7572) (71.8965, -26.6153) (72.9348, -26.451) (73.3531, -26.451) knots 0 0 0 1 2 2 2
  spline S208 degree 2 poles (73.3531, -26.451) (74.6155, -26.451) (76.0049, -27.5415) (76.0049, -28.4827) knots 0 0 0 1 2 2 2
  line L123 (76.0049, -28.4827) -> (76.0049, -31.2614)
  line L124 (76.0049, -31.2614) -> (76.2364, -31.2614)
  spline S209 degree 2 poles (76.2364, -31.2614) (76.7444, -31.2614) (77.1627, -31.6349) (77.1627, -31.9412) knots 0 0 0 1 2 2 2
  spline S210 degree 2 poles (77.1627, -31.9412) (77.1627, -32.2474) (76.7444, -32.6134) (76.2364, -32.6134) knots 0 0 0 1 2 2 2
  line L125 (76.2364, -32.6134) -> (74.6528, -32.6134)
  spline S211 degree 2 poles (74.6528, -30.1933) (73.8461, -30.0364) (73.1589, -30.0364) knots 0 0 0 1 1 1
  spline S212 degree 2 poles (73.1589, -30.0364) (72.3373, -30.0364) (71.7397, -30.4398) knots 0 0 0 1 1 1
  spline S213 degree 2 poles (71.7397, -30.4398) (71.3737, -30.6937) (71.3737, -30.9552) knots 0 0 0 1 1 1
  spline S214 degree 2 poles (71.3737, -30.9552) (71.3737, -31.1419) (71.5529, -31.2614) knots 0 0 0 1 1 1
  spline S215 degree 2 poles (71.5529, -31.2614) (71.8816, -31.478) (72.4568, -31.478) knots 0 0 0 1 1 1
  spline S216 degree 2 poles (72.4568, -31.478) (72.9423, -31.478) (74.1748, -31.0971) (74.6528, -30.7684) knots 0 0 0 1 2 2 2
  line L126 (74.6528, -30.7684) -> (74.6528, -30.1933)
  point P0 (-10, -21.48)
  constraints: 2 other
extrude "Extrusion7" add sketch "Sketch9" along normal blind 2
body "Solid1"
